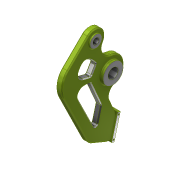
# Autodesk Inventor part: 1_Crusher_Arm
Saved by Autodesk Inventor 2020.1 (Build 241239000, 239)
## iProperties
Part Number: 1_Crusher_Arm
Document SubType Name: Modeling
Created: 2003-02-27
Material: Standard
Designer: Joe M
Engineer: Joe M
Density: 1 g/cm^3
Appearance: Canary
Control State: 0
Master: False
Checked Out: False
Shininess: 64.0
Length Units: 11269
Angle Units: 11279
Time Units: 11290
Mass Units: 11283
Length Display Precision: 3
Angle Display Precision: 2
Compacted: True
d98: 100.000 mm
d96: 2.000 ul
Density: 0.0
Volumn: 0.0
Area: 0.0
PropertySet Name: Model Information
Author: Joe M
Autodesk Inventor part; units mm, degrees
ref_plane "YZ Plane" through (0, 0, 0) normal (1, 0, 0) x (0, 1, 0)
ref_plane "XZ Plane" through (0, 0, 0) normal (0, 1, 0) x (-1, 0, 0)
ref_plane "XY Plane" through (0, 0, 0) normal (0, 0, 1) x (1, 0, 0)
sketch "Skizze1" plane through (0, 0, 0) normal (0, 0, 1) x (1, 0, 0)
  circle A0 centre (0, 0) radius 25 construction
  circle A1 centre (-75.603, 171.4328) radius 15
  circle A2 centre (0, 0) radius 50
  circle A3 centre (-75.603, 171.4328) radius 30
  circle A4 centre (-75.603, 171.4328) radius 50
  arc A5 (24.9981, -65.3842) -> (5.7804, 69.7609) centre (0, 0) ccw
  line L0 (0, 0) -> (0, -250)
  circle A6 centre (0, -250) radius 50
  arc A7 (-32.8469, 145.5115) -> (5.7804, 69.7609) centre (9.9092, 119.5902) ccw
  line L1 (-19.196, -296.1683) -> (-88.6853, -267.2759)
  arc A8 (-114.3423, -243.2032) -> (-88.6853, -267.2759) centre (-69.4894, -221.1076) ccw
  line L2 (-114.3423, -243.2032) -> (-230.6222, -7.1613)
  arc A9 (-211.0499, 108.3131) -> (-230.6222, -7.1613) centre (-140.9164, 37.0299) ccw
  line L3 (-211.0499, 108.3131) -> (-110.6698, 207.0743)
  line L4 (45.8258, -230) -> (0, -125)
  arc A10 (24.9981, -65.3842) -> (0, -125) centre (40.9568, -107.125) ccw
  line L5 (0, 0) -> (-211.0499, 108.3131) construction
  line L6 (-75.603, 171.4328) -> (-129.4808, 66.4509) construction
  dimension "d1" = 50
  dimension "d2" = 30
  dimension "d3" = 100
  dimension "d4" = 60
  dimension "d5" = 100
  dimension "d25" = 250
  dimension "d26" = 50
  dimension "d41" = 70
  dimension "d101" = 100
  dimension "d103" = 50
  dimension "d104" = 26.226
  dimension "d116" = 118
  constraints: 14 end point, 14 point on circle, 11 centre point, 11 tangent, 4 coincident, 2 concentric, 1 equal radius, 1 midpoint, 1 perpendicular, 1 point on line, 1 vertical alignment, 1 other
  measures "d1" diameter of A0
  measures "d2" diameter of A1
  measures "d3" diameter of A2
  measures "d4" diameter of A3
  measures "d5" diameter of A4
  measures "d25" distance of L0.end point (0, 0)
  measures "d26" radius of A7
  measures "d41" radius of A5
  measures "d101" radius of A9
  measures "d103" radius of A8
  measures "d104" angle of L0 L2
  measures "d116" distance of L6.start L6.end
extrude "Extrusion1" add sketch "Skizze1" against normal mid plane 30 contours A1 | A2 | A3 | A4 | A4 A7 A5 A10 L0 A6 L1 A8 L2 A9 L3 | L4 A6 L0 | A6
extrude "Extrusion2" add sketch "Skizze1" against normal mid plane 60 contours A2
extrude "Extrusion3" add sketch "Skizze1" along normal mid plane 40 contours A1 | A3
extrude "Extrusion4" cut sketch "Skizze1" along normal through all both and the other way through all contours A1
sketch "Skizze3" plane through (0, 0, 15) normal (0, 0, 1) x (1, 0, 0)
  line L0 (31.3652, -196.8667) -> (4.4712, -299.7997)
  line L1 (0, -125) -> (45.8258, -230) projected
  arc A0 (-19.196, -296.1683) -> (45.8258, -230) centre (0, -250) ccw projected
  constraints: 2 end point, 1 point on circle, 1 point on line, 1 other
extrude "Extrusion6" cut sketch "Skizze3" against normal through all
sketch "Skizze13" plane through (4.4712, -299.7997, 15) normal (0.9675208, -0.2527914, 0) x (0, 0, -1)
  line L0 (-5, 113.1942) -> (35, 113.1942)
  line L1 (35, 113.1942) -> (35, -6.8058)
  line L2 (35, -6.8058) -> (-5, -6.8058)
  line L3 (-5, -6.8058) -> (-5, 113.1942)
  line L4 (0, 0) -> (0, 106.3884) projected
  point P0 (15, 113.1942)
  point P1 (-5, 53.1942)
  point P2 (0, 53.1942)
  dimension "d75" = 40
  dimension "d76" = 120
  constraints: 8 end point, 3 midpoint, 2 parallel, 1 horizontal, 1 horizontal alignment, 1 perpendicular
  measures "d75" distance of L0.start L0.end
  measures "d76" distance of L2.end L0.start
extrude "Extrusion16" add sketch "Skizze13" along normal blind 15
sketch "Skizze15" plane through (0, 0, 15) normal (0, 0, 1) x (1, 0, 0)
  line L0 (4.4712, -299.7997) -> (31.3652, -196.8667) projected
  line L1 (0, -125) -> (31.3652, -196.8667) projected
  line L2 (-114.3423, -243.2032) -> (-230.6222, -7.1613) projected
  line L3 (-178.4123, 0) -> (-69.4894, -221.1076)
  line L4 (-69.4894, -221.1076) -> (-44.1034, -123.9465)
  line L5 (-44.1034, -123.9465) -> (-98.1981, 0)
  arc A0 (-114.3423, -243.2032) -> (-88.6853, -267.2759) centre (-69.4894, -221.1076) ccw projected
  arc A1 (24.9981, -65.3842) -> (5.7804, 69.7609) centre (0, 0) ccw projected
  line L6 (-211.0499, 108.3131) -> (-110.6698, 207.0743) projected
  circle A2 centre (0, 0) radius 50 projected
  line L7 (-95.0087, 24.8236) -> (-172.6176, 45.1011)
  line L8 (2.7507, -306.3845) -> (33.0857, -190.282) projected
  line L9 (-178.4123, 0) -> (-98.1981, 0)
  line L10 (0, 0) -> (-178.4123, 0) construction
  circle A3 centre (0, 0) radius 98.1981 construction
  circle A4 centre (0, 0) radius 178.4123 construction
  line L11 (0, 0) -> (-68.8698, 69.9987) construction
  line L12 (-68.8698, 69.9987) -> (-125.1269, 127.1779)
  line L13 (-172.6176, 45.1011) -> (-125.1269, 127.1779)
  line L14 (-95.0087, 24.8236) -> (-68.8698, 69.9987)
  point P0 (8.6917, 119.6848)
  dimension "d107" = 40
  constraints: 21 end point, 6 point on circle, 4 parallel, 2 centre point, 2 coincident, 2 perpendicular, 2 point on line, 1 collinear, 1 horizontal
  measures "d107" distance between parallel lines of L1 L5
extrude "Extrusion17" cut sketch "Skizze15" against normal through all contours L9 L5 L4 L3 | L7 L13 L12 L14
fillet "Rundung9" radius 30 3 edges at (-178.4123, 0, 0) (-125.1269, 127.1779, 0) (-172.6176, 45.1011, 0)
fillet "Rundung9" radius 10 5 edges at (-44.1034, -123.9465, 0) (-98.1981, 0, 0) (-69.4894, -221.1076, 0) (-95.0087, 24.8236, 0) (-68.8698, 69.9987, 0)
chamfer "Chamfer3" distance 5 angle 45 32 edges at (-119.2264, -120.144, 15) (-155.6636, -14.1526, 15) (-117.4677, 0, 15) (-99.2674, -1.6334, 15) (-70.5344, -63.3855, 15) (-44.6848, -123.9919, 15) (-53.8419, -161.2191, 15) (-71.3706, -202.5604, 15) (-70.5344, -63.3855, -15) (-99.2674, -1.6334, -15) (-117.4677, 0, -15) (-155.6636, -14.1526, -15) (-119.2264, -120.144, -15) (-71.3706, -202.5604, -15) (-53.8419, -161.2191, -15) (-44.6848, -123.9919, -15) (-81.9392, 47.4111, 15) (-95.9985, 27.1955, 15) (-118.4429, 30.9465, 15) (-154.6103, 52.6158, 15) (-148.8722, 86.1395, 15) (-122.6678, 107.821, 15) (-85.8567, 87.2641, 15) (-71.4195, 69.6747, 15) (-85.8567, 87.2641, -15) (-122.6678, 107.821, -15) (-148.8722, 86.1395, -15) (-154.6103, 52.6158, -15) (-118.4429, 30.9465, -15) (-95.9985, 27.1955, -15) (-81.9392, 47.4111, -15) (-71.4195, 69.6747, -15)
fillet "Rundung11" radius 5 4 edges at (-105.603, 171.4328, 15) (-50, 0, 15) (-50, 0, -15) (-105.603, 171.4328, -15)
sketch "Skizze16" plane through (2.7507, -306.3845, 20) normal (0, 0, 1) x (0.9675208, -0.2527914, 0)
  line L0 (0, 120) -> (15, 120) projected
  point P0 (7.5, 110)
  point P1 (7.5, 120)
  dimension "d88" = 10
  constraints: 1 midpoint, 1 vertical alignment
  measures "d88" distance from line of L0 point (7.5, 110)
hole "Bohrung2" at (37.8142, -201.8531, 20) direction (0, 0, -1) diameter 6.647 end through all thread size "M8x1.25" class "6H" standard "ISO Metrisches Profil"
pattern_linear "Rechteckige Anordnung1" count 2 spacing 100 along (-0.2527914, -0.9675208, 0) of "Bohrung2"
chamfer "Fase1" distance 2 angle 45 2 edges at (32.431, -252.1251, 20) (32.431, -252.1251, -20)
chamfer "Chamfer2" distance 5 angle 45 22 edges at (-160.8598, 157.6937, 15) (-44.5824, 210.6466, 15) (-34.6338, 96.8764, 15) (69.3028, 9.8549, 15) (-0.2543, -89.8443, 15) (15.6826, -160.9334, 15) (-239.5102, 53.741, 15) (-172.4822, -125.1823, 15) (-103.701, -257.5707, 15) (-53.9407, -281.7221, 15) (-7.583, -299.4216, 15) (-160.8598, 157.6937, -15) (-239.5102, 53.741, -15) (-172.4822, -125.1823, -15) (-103.701, -257.5707, -15) (-53.9407, -281.7221, -15) (-7.583, -299.4216, -15) (-44.5824, 210.6466, -15) (-34.6338, 96.8764, -15) (69.3028, 9.8549, -15) (-0.2543, -89.8443, -15) (15.6826, -160.9334, -15)
hole "Hole3" at (0, 0, 30) direction (0, 0, -1) diameter 50 end through all
body "Solid1"
